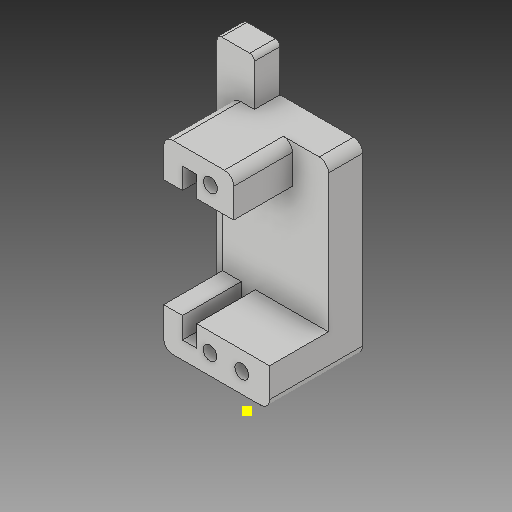
# Autodesk Inventor part: SyringeMotorBase
Saved by Autodesk Inventor 2018 (Build 220112000, 112)
## iProperties
Created: 2018-05-20
Part Number: SyringeMotorBase
Material: Generic
Document SubType Name: Modeling
Designer: reide
Density: 1 g/cm^3
Appearance: Default
Author: reide
Autodesk Inventor part; units mm, degrees
sketch "Sketch1" plane through (0, 0, 0) normal (0, 0, 1) x (1, 0, 0)
  line L0 (4.9653, 56.3387) -> (16.6724, 56.3387) projected
  line L1 (4.9653, 56.3387) -> (4.9653, 55.3387)
  line L2 (17.6724, 57.3387) -> (17.6724, 77.3387) projected
  line L3 (17.6724, 55.3387) -> (-12.3276, 55.3387)
  line L4 (-12.3276, 55.3387) -> (-12.3276, 15.3387)
  line L5 (-12.3276, 15.3387) -> (17.6724, 15.3387)
  line L6 (17.6724, 15.3387) -> (17.6724, 55.3387)
  point P0 (0, 0)
  dimension "d0" = 1
  dimension "d1" = 40
  dimension "d2" = 0
  dimension "d3" = 30
  dimension "d4" = 0
  constraints: 10 end point, 2 parallel, 1 horizontal, 1 perpendicular, 1 vertical
  measures "d0" distance of L0.start L1.end
  measures "d1" distance between parallel lines of L5 L3
  measures "d2" distance from line of L3 L1.end
  measures "d3" distance of L4.end L5.end
  measures "d4" distance between parallel lines of L2 L6
ref_plane "Work Plane1" through (-14.696, -74.3472, 7.3936) normal (0, 0, 1) x (1, 0, 0)
extrude "Extrusion1" add sketch "Sketch1" along normal up to surface (7.3936 mm away)
sketch "Sketch2" plane through (-12.3276, 15.3387, 0) normal (-1, 0, 0) x (0, 0, 1)
  line L0 (0, 18.6738) -> (12.7, 18.6738) projected
  line L1 (7.3936, 0) -> (7.3936, 40) projected
  line L2 (0, 40) -> (7.3936, 40) projected
  line L3 (0, 40) -> (0, 0) projected
  line L4 (0, 0) -> (7.3936, 0) projected
  point P0 (0, -15.3387)
ref_plane "Work Plane2" through (-5.1876, 23.3419, 7.3936) normal (-1, 0, 0) x (0, 0, 1)
extrude "Extrusion2" cut sketch "Sketch2" against normal up to surface (7.14 mm away)
sketch "Sketch3" plane through (0, 0, 0) normal (0, 0, -1) x (-1, 0, 0)
  line L0 (-17.6724, 55.3387) -> (5.1876, 55.3387) projected
  line L1 (5.1876, 55.3387) -> (1.1876, 55.3387)
  line L2 (1.1876, 55.3387) -> (1.1876, 51.3387)
  circle A0 centre (1.1876, 51.3387) radius 1.625
  line L3 (5.1876, 55.3387) -> (5.1876, 15.3387) projected
  line L4 (5.1876, 35.3387) -> (-17.6724, 35.3387)
  line L5 (-6.2424, 55.3387) -> (-6.2424, 15.3387)
  line L6 (1.1876, 15.3387) -> (1.1876, 19.3387)
  circle A1 centre (1.1876, 19.3387) radius 1.625
  line L7 (5.1876, 55.3387) -> (-17.6724, 55.3387)
  line L8 (-17.6724, 55.3387) -> (-13.6724, 55.3387)
  line L9 (-13.6724, 55.3387) -> (-13.6724, 51.3387)
  circle A2 centre (-13.6724, 51.3387) radius 1.625
  line L10 (-17.6724, 55.3387) -> (-17.6724, 15.3387)
  line L11 (-17.6724, 35.3387) -> (5.1876, 35.3387)
  line L12 (-13.6724, 15.3387) -> (-13.6724, 19.3387)
  circle A3 centre (-13.6724, 19.3387) radius 1.625
  point P0 (0, 0)
  dimension "d9" = 4
  dimension "d10" = 4
  dimension "d11" = 3.25
  constraints: 22 end point, 14 symmetric about line, 4 centre point, 4 coincident, 2 midpoint, 2 point on line, 1 horizontal, 1 perpendicular, 1 vertical, 3 other
  measures "d9" distance of L0.end L1.end
  measures "d10" distance of L1.end L2.end
  measures "d11" diameter of A0
extrude "Extrusion3" cut sketch "Sketch3" against normal blind 5 contours A0 | A1 | A2 | A3
fillet "Fillet1" radius 2 4 edges at (17.6724, 55.3387, 3.6968) (-5.1876, 55.3387, 3.6968) (17.6724, 15.3387, 3.6968) (-5.1876, 15.3387, 3.6968)
sketch "Sketch4" plane through (-3.1876, 15.3387, 7.3936) normal (0, 0, 1) x (1, 0, 0)
  point P0 (3.1876, -15.3387)
sketch "Sketch5" plane through (-3.1876, 15.3387, 7.3936) normal (0, 0, 1) x (1, 0, 0)
  line L0 (13.108, 31.43) -> (13.108, 40) projected
  line L1 (13.108, 40) -> (0, 40) projected
  arc A0 (0, 40) -> (-2, 38) centre (0, 38) ccw projected
  line L2 (-2, 38) -> (-2, 2) projected
  arc A1 (-2, 2) -> (0, 0) centre (0, 2) ccw projected
  line L3 (0, 0) -> (18.86, 0) projected
  arc A2 (18.86, 0) -> (20.86, 2) centre (18.86, 2) ccw projected
  line L4 (20.86, 2) -> (20.86, 31.43) projected
  line L5 (20.86, 31.43) -> (13.108, 31.43) projected
  line L6 (5.108, 36.252) -> (2.068, 36.252) projected
  line L7 (5.108, 31.68) -> (5.108, 36.252) projected
  line L8 (2.068, 36.252) -> (2.068, 31.68) projected
  line L9 (13.108, 31.68) -> (5.108, 31.68) projected
  line L10 (2.068, 31.68) -> (-2, 31.68) projected
  line L11 (6.0288, 20) -> (-2, 20)
  line L12 (-2, 2) -> (-2, 38) projected
  line L13 (13.108, 8.57) -> (13.108, 0)
  line L14 (13.108, 0) -> (0, 0)
  arc A3 (-2, 2) -> (0, 0) centre (0, 2) ccw
  line L15 (-2, 2) -> (-2, 38)
  line L16 (20.86, 8.57) -> (13.108, 8.57)
  line L17 (5.108, 3.748) -> (2.068, 3.748)
  line L18 (5.108, 8.32) -> (5.108, 3.748)
  line L19 (2.068, 3.748) -> (2.068, 8.32)
  line L20 (13.108, 8.32) -> (5.108, 8.32)
  line L21 (2.068, 8.32) -> (-2, 8.32)
  line L22 (-2, 38) -> (-2, 2)
  line L23 (13.108, 8.32) -> (20.86, 8.32)
  line L24 (20.86, 8.32) -> (20.86, 2)
  line L25 (18.86, 0) -> (13.108, 0)
  line L26 (13.108, 0) -> (13.108, 8.32)
  arc A4 (18.86, 0) -> (20.86, 2) centre (18.86, 2) ccw
  point P0 (0, 2)
  dimension "d21" = 2
  constraints: 30 end point, 12 symmetric about line, 4 point on circle, 2 centre point, 2 parallel, 2 tangent, 1 horizontal, 1 midpoint, 1 perpendicular, 1 other
  measures "d21" radius of A4
ref_plane "Work Plane3" through (-5.1876, 19.3367, 20.0936) normal (0, 0, 1) x (1, 0, 0)
extrude "Extrusion4" add sketch "Sketch5" along normal up to surface (12.7 mm away) contours L9 L7 L6 L8 L10 L2 A0 L1 L0 | L4 A2 L3 L13 L23 | L13 L3 A1 L2 L21 L19 L17 L18 L20
sketch "Sketch6" plane through (-3.1876, 55.3387, 20.0936) normal (0, 0, 1) x (1, 0, 0)
  line L0 (0, -40) -> (18.86, -40) projected
  circle A0 centre (14.86, -35.715) radius 1.75 projected
  circle A1 centre (8.108, -4.285) radius 1.75 projected
  circle A2 centre (8, -35.715) radius 1.75 projected
  circle A3 centre (8.108, -4.285) radius 1.5
  circle A4 centre (8, -35.715) radius 1.5
  circle A5 centre (14.86, -35.715) radius 1.5
  line L1 (12.108, -2) -> (12.108, -9.57) projected
  arc A6 (12.108, -2) -> (11.108, -1) centre (11.108, -2) ccw projected
  line L2 (0, -1) -> (11.108, -1) projected
  arc A7 (0, -1) -> (-1, -2) centre (0, -2) ccw projected
  line L3 (-1, -38) -> (-1, -2) projected
  arc A8 (-1, -38) -> (0, -39) centre (0, -38) ccw projected
  line L4 (18.86, -39) -> (0, -39) projected
  arc A9 (18.86, -39) -> (19.86, -38) centre (18.86, -38) ccw projected
  line L5 (19.86, -10.57) -> (19.86, -38) projected
  arc A10 (19.86, -10.57) -> (18.86, -9.57) centre (18.86, -10.57) ccw projected
  line L6 (12.108, -9.57) -> (18.86, -9.57) projected
  point P0 (3.1876, -55.3387)
  dimension "d24" = 3
  dimension "d25" = 3
  dimension "d26" = 3
  constraints: 3 centre point, 3 coincident
  measures "d24" diameter of A3
  measures "d25" diameter of A4
  measures "d26" diameter of A5
extrude "Extrusion5" cut sketch "Sketch6" against normal blind 7 contours A3 | A4 | A5
fillet "Fillet2" radius 2 1 edges at (9.9204, 55.3387, 13.7436)
sketch "Sketch7" plane through (0, 0, 0) normal (0, 0, -1) x (-1, 0, 0)
  line L0 (8.5531, 55.2077) -> (8.5531, 16.3387) projected
  line L1 (5.1876, 15.3387) -> (8.2876, 15.3387)
  line L2 (5.1876, 15.3387) -> (8.2876, 15.3387)
  line L3 (3.1876, 15.3387) -> (-15.6724, 15.3387) projected
  line L4 (5.1876, 15.3387) -> (3.1876, 15.3387)
  arc A0 (-7.9204, 55.3387) -> (-9.9204, 53.3387) centre (-7.9204, 53.3387) ccw projected
  line L5 (3.1876, 55.3387) -> (-7.9204, 55.3387) projected
  arc A1 (5.1876, 53.3387) -> (3.1876, 55.3387) centre (3.1876, 53.3387) ccw projected
  line L6 (5.1876, 47.0187) -> (5.1876, 53.3387) projected
  line L7 (1.1196, 47.0187) -> (5.1876, 47.0187) projected
  line L8 (1.1196, 51.5907) -> (1.1196, 47.0187) projected
  line L9 (-1.9204, 51.5907) -> (1.1196, 51.5907) projected
  line L10 (-1.9204, 47.0187) -> (-1.9204, 51.5907) projected
  line L11 (-9.9204, 47.0187) -> (-1.9204, 47.0187) projected
  line L12 (-9.9204, 53.3387) -> (-9.9204, 47.0187) projected
  circle A2 centre (-4.9204, 51.0537) radius 1.5 projected
  line L13 (3.1876, 15.3387) -> (5.1876, 15.3387)
  line L14 (5.1876, 15.3387) -> (5.1876, 55.3387)
  line L15 (5.1876, 55.3387) -> (3.1876, 55.3387)
  line L16 (3.1876, 55.3387) -> (3.1876, 15.3387)
  line L17 (0.1876, 55.3387) -> (5.1876, 55.3387)
  line L18 (5.1876, 55.3387) -> (8.2876, 55.3387)
  line L19 (3.2876, 15.3387) -> (8.2876, 15.3387)
  line L20 (8.2876, 15.3387) -> (5.1876, 15.3387)
  line L21 (5.1876, 15.3387) -> (5.1876, 55.3387)
  line L22 (5.1876, 55.3387) -> (8.2876, 55.3387)
  line L23 (8.2876, 55.3387) -> (8.2876, 15.3387)
  line L24 (3.1876, 55.3387) -> (5.1876, 55.3387)
  line L25 (5.1876, 55.3387) -> (5.1876, 15.3387)
  line L26 (5.1876, 15.3387) -> (3.1876, 15.3387)
  line L27 (3.1876, 15.3387) -> (3.1876, 55.3387)
  line L28 (8.2876, 15.3387) -> (8.2876, 65.3387)
  line L29 (8.2876, 15.3387) -> (5.1876, 15.3387)
  line L30 (5.1876, 15.3387) -> (5.1876, 65.3387)
  line L31 (5.1876, 65.3387) -> (8.2876, 65.3387)
  line L32 (8.2876, 65.3387) -> (8.2876, 15.3387)
  line L33 (3.1876, 55.3387) -> (5.1876, 55.3387)
  line L34 (5.1876, 55.3387) -> (5.1876, 15.3387)
  line L35 (5.1876, 15.3387) -> (3.1876, 15.3387)
  line L36 (3.1876, 15.3387) -> (3.1876, 55.3387)
  line L37 (5.1876, 55.3387) -> (0.1876, 55.3387)
  line L38 (-15.6724, 55.3387) -> (3.1876, 55.3387) projected
  line L39 (0.1876, 55.3387) -> (5.1876, 55.3387)
  line L40 (5.1876, 55.3387) -> (5.1876, 65.3387)
  line L41 (5.1876, 65.3387) -> (0.1876, 65.3387)
  line L42 (0.1876, 65.3387) -> (0.1876, 55.3387)
  point P0 (0, 0)
  dimension "d30" = 3.1
  dimension "d39" = 50
  dimension "d40" = 5
  constraints: 64 end point, 12 parallel, 9 horizontal, 8 perpendicular, 3 point on line, 1 collinear, 1 point on circle
  measures "d30" distance of L1.start L1.end
  measures "d39" distance of L19.end L28.end
  measures "d40" distance of L33.end L17.start
ref_plane "Work Plane4" through (-18.3321, 13.5596, 5.5) normal (0, 0, 1) x (1, 0, 0)
extrude "Extrusion6" add sketch "Sketch7" against normal up to surface (5.5 mm away) contours L14 L6 L18 L23 L1 | L4 L16 L7 L14 | L7 L16 A1 L6 | L18 L30 L31 L28 | A1 L15 L14 | L15 L5 L42 L41 L30 | A2
fillet "Fillet3" radius 1 3 edges at (-8.2876, 65.3387, 2.75) (-0.1876, 65.3387, 2.75) (-8.2876, 15.3387, 2.75)
body "Solid1"
